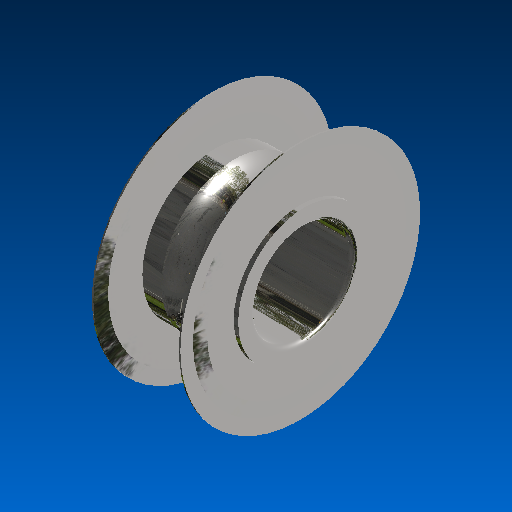
# Autodesk Inventor part: W 606-2Z_PART1
Saved by Autodesk Inventor 2018 (Build 220112000, 112)
## iProperties
Category: PARTsolutions
Company: SKF
Part Number: W 606-2Z_PART1
Material: Stainless Steel
Catalog Web Link: www.cadenas.de
Description: -Deep groove ball bearings
Vendor: SKF
Document SubType Name: Modeling
Designer: partserver
Manufacturer: SKF
Mass: 1.63715 g
Surface Area: 8.25973 cm^2
Volume: 0.204644 cm^3
Density: 8 g/cm^3
Appearance: Semi-Polished
PSOL_IDENT_0: {$CADENAS_DATA\23d-libs\skf_r32\bearings_units_and_housings\ball_bearings\deep_groove_ball_bearings\
PSOL_IDENT_1: bb1_001_101.prj},195 {VTYP=3D},{NB=W 606-2Z_PART1},{LINA=W 606-2Z_PART1},{NN=BB1_001_101_PART1},{NOP
PSOL_IDENT_2: RJ=TRUE},{DATE=10.06.2020 10:28:41},{GEOMDATE=07.04.2020 07:08:50},{VERSION=},{LINEID=16750},{WBVAR=
PSOL_IDENT_3: },{WBNUMERIC=}  {NB=W 606-2Z_PART1},{LINA=W 606-2Z_PART1},{KT=DUMMY},{DESIGNATION=W 606-2Z},{DD=6.00
PSOL_IDENT_4: 0},{D=17.000},{B=6.000},{C=0.000},{DD1=0.00},{DD2=8.20},{D1=0.00},{D2=14.80},{D3=0.000},{D4=0.000},{
PSOL_IDENT_5: HH=MIN},{BB=0.000},{FF=0.00},{R0MAX=MIN},{R0=MIN},{R12=0.30},{PITCH=11.30},{DW=3.500},{DDAMIN=7.700}
PSOL_IDENT_6: ,{DDAMAX=8.100},{DDBMIN=MIN},{DDBMAX=MIN},{DBMIN=MIN},{DAMAX=15.000},{BBAMIN=MIN},{CAMAX=MIN},{RAMAX=
PSOL_IDENT_7: 0.300},{LOAD1=1.950},{LOAD2=0.830},{LOAD3=0.036},{SPEED1=95000},{SPEED2=48000},{KR=0.030},{F0=11.400
PSOL_IDENT_8: },{Z=6},{II=1},{MASS=0.006},{BEARING=W 606-2Z},{RING=},{HELP=1.677},{HELP2=1.100},{DD1ALG=3.900},{YA
PSOL_IDENT_9: LG=4.513},{PITCH1=11.300},{DW1=3.500},{YALG1=6.823},{HALG1=1.677},{SH=4.100},{CU=0.500},{DESIGN=dgbb
PSOL_IDENT_10: w2z},{HALG=1.5125},{B1=0},{SHIELDHELP=2}
NB: W 606-2Z_PART1
NT: Deep groove ball bearings
NBSYN: $DESIGNATION._PART1
LINA: W 606-2Z_PART1
CATALOG: SKF
SUPPLIER: SKF
ARTICLENO: W 606-2Z_PART1
BOMINFO: W 606-2Z_PART1
CREATOR: CADENAS GmbH
Title: W 606-2Z_PART1
Author: Cadenas PARTsolutions
Comments: Deep groove ball bearings
Autodesk Inventor part; units mm, degrees
ref_plane "YZ Plane" through (0, 0, 0) normal (1, 0, 0) x (0, 1, 0)
ref_plane "XZ Plane" through (0, 0, 0) normal (0, 1, 0) x (-1, 0, 0)
ref_plane "XY Plane" through (0, 0, 0) normal (0, 0, 1) x (1, 0, 0)
sketch "Sketch_18" plane through (0, 0, 0) normal (0, 0, 1) x (1, 0, 0)
  line L0 (50, 0) -> (-50, 0)
  arc A0 (0, 3.3005) -> (0.3, 3.0005) centre (0.3, 3.3005) ccw
  line L1 (0.3, 3.0005) -> (5.7, 3.0005)
  arc A1 (5.7, 3.0005) -> (6, 3.3005) centre (5.7, 3.3005) ccw
  line L2 (6, 3.3005) -> (6, 4.513)
  line L3 (6, 4.513) -> (4.3303, 4.513)
  arc A2 (1.6697, 4.513) -> (4.3303, 4.513) centre (3, 5.65) ccw
  line L4 (1.6697, 4.513) -> (0, 4.513)
  line L5 (0, 4.513) -> (0, 3.3005)
  constraints: 12 end point, 6 point on circle, 3 centre point
revolve "Revolution1" add sketch "Sketch_18" angle 360 about axis through (50, 0, 0) along (1, 0, 0)
sketch "Sketch_19" plane through (0, 0, 0) normal (0, 0, 1) x (1, 0, 0)
  line L0 (50, 0) -> (-50, 0)
  line L1 (0, 5.5125) -> (0, 4.1)
  line L2 (0, 4.1) -> (0.2917, 4.1)
  arc A0 (0.2917, 4.1) -> (0.5, 4.3083) centre (0.2917, 4.3083) ccw
  line L3 (0.5, 4.3083) -> (0.5, 5.1792)
  line L4 (0.5, 5.1792) -> (5.5, 5.1792)
  line L5 (5.5, 5.1792) -> (5.5, 4.3083)
  arc A1 (5.5, 4.3083) -> (5.7083, 4.1) centre (5.7083, 4.3083) ccw
  line L6 (5.7083, 4.1) -> (6, 4.1)
  line L7 (6, 4.1) -> (6, 5.5125)
  line L8 (6, 5.5125) -> (0, 5.5125)
  constraints: 18 end point, 4 point on circle, 2 centre point
revolve "Revolution2" cut sketch "Sketch_19" angle 360 about axis through (50, 0, 0) along (1, 0, 0)
sketch "Sketch_20" plane through (0, 0, 0) normal (0, 0, 1) x (1, 0, 0)
  line L0 (50, 0) -> (-50, 0)
  line L1 (0.27, 7.4) -> (0.315, 6.5725)
  line L2 (0.315, 6.5725) -> (0.27, 5.745)
  line L3 (0.27, 5.745) -> (0.27, 4.09)
  line L4 (0.27, 4.09) -> (0.36, 4.09)
  line L5 (0.36, 4.09) -> (0.45, 5.745)
  line L6 (0.45, 5.745) -> (0.45, 6.5725)
  line L7 (0.45, 6.5725) -> (0.36, 7.4)
  line L8 (0.36, 7.4) -> (0.27, 7.4)
  constraints: 18 end point
revolve "Revolution3" add sketch "Sketch_20" angle 360 about axis through (50, 0, 0) along (1, 0, 0)
sketch "Sketch_21" plane through (0, 0, 0) normal (0, 0, 1) x (1, 0, 0)
  line L0 (50, 0) -> (-50, 0)
  line L1 (5.55, 6.5725) -> (5.55, 5.745)
  line L2 (5.55, 5.745) -> (5.64, 4.09)
  line L3 (5.64, 4.09) -> (5.73, 4.09)
  line L4 (5.73, 4.09) -> (5.73, 5.745)
  line L5 (5.73, 5.745) -> (5.685, 6.5725)
  line L6 (5.685, 6.5725) -> (5.73, 7.4)
  line L7 (5.73, 7.4) -> (5.64, 7.4)
  line L8 (5.64, 7.4) -> (5.55, 6.5725)
  constraints: 18 end point
revolve "Revolution4" add sketch "Sketch_21" angle 360 about axis through (50, 0, 0) along (1, 0, 0)
body "Solid1"
